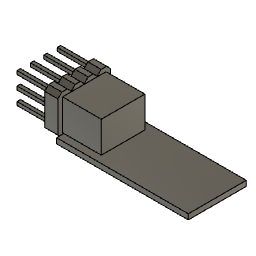
_FS2A Receiver.9ec7e849-6926-4f4f-884d-18c81e3adff5 (Autodesk Fusion 360 design; units mm, degrees)
Autodesk Fusion 360 part; units mm, degrees
sketch "Sketch1" plane through (0, 0, 0) normal (0, 0, 1) x (1, 0, 0)
  line L0 (-12.5, 5.5) -> (12.5, 5.5)
  line L1 (12.5, 5.5) -> (12.5, -5.5)
  line L2 (12.5, -5.5) -> (-12.5, -5.5)
  line L3 (-12.5, -5.5) -> (-12.5, 5.5)
  line L4 (-12.5, 5.5) -> (12.5, -5.5) construction
  line L5 (12.5, 5.5) -> (-12.5, -5.5) construction
  line L6 (-12.5, 5.5) -> (-21.5, 5.5) construction
  line L7 (-21.5, 5.5) -> (-21.5, -5.5) construction
  line L8 (-21.5, -5.5) -> (-12.5, -5.5) construction
  dimension "d1" = 11
  dimension "d2" = 25
  dimension "d5" = 34
  constraint horizontal L0
  constraint vertical L1
  constraint horizontal L2
  constraint vertical L3
  constraint coincident origin L5
  constraint coincident origin L4
  constraint perpendicular L3 L6
  constraint perpendicular L2 L7
  constraint perpendicular L3 L8
  measures "d1" distance of L0.start L2.end
  measures "d2" distance of L0.start L0.end
  measures "d5" distance of L1 L7
extrude "Extrude1" add sketch "Sketch1" along normal blind 1 makes body 1
sketch "Sketch2" plane through (0, 0, 0) normal (0, 1, 0) x (1, 0, 0)
  line L0 (-15.25, -7.75) -> (-12.75, -7.75)
  line L1 (-12.75, -7.75) -> (-12.75, -0.31)
  line L2 (-12.75, -0.31) -> (-15.25, -0.31)
  line L3 (-15.25, -0.31) -> (-15.25, -7.75)
  point P0 (12.5, 0)
  dimension "d6" = 2.5
  dimension "d7" = 7.44
  dimension "d8" = 7.75
  dimension "d9" = 27.75
  constraint horizontal L0
  constraint perpendicular L0 L1
  constraint perpendicular L1 L2
  constraint perpendicular L0 L3
  constraint coincident L0.start L3.end
  measures "d6" distance of L0.start L0.end
  measures "d7" distance of L2.end L0.start
  measures "d8" distance of origin L0
  measures "d9" distance of L3 P0
extrude "Extrude2" add sketch "Sketch2" along normal mid plane 10 separate body makes body 2
sketch "Sketch3" plane through (-15.25, 0, 0) normal (-1, 0, 0) x (0, -1, 0)
  line L0 (5, 7.75) -> (-5, 7.75)
  line L1 (-5, 7.75) -> (-5, 0.31)
  line L2 (-5, 0.31) -> (5, 0.31)
  line L3 (5, 0.31) -> (5, 7.75)
  line L4 (-4.15, 6.9) -> (-3.5, 6.9)
  line L5 (-3.5, 6.9) -> (-3.5, 6.25)
  line L6 (-3.5, 6.25) -> (-4.15, 6.25)
  line L7 (-4.15, 6.25) -> (-4.15, 6.9)
  line L8 (-1.61, 6.9) -> (-0.96, 6.9)
  line L9 (-0.96, 6.9) -> (-0.96, 6.25)
  line L10 (-0.96, 6.25) -> (-1.61, 6.25)
  line L11 (-1.61, 6.25) -> (-1.61, 6.9)
  line L12 (0.93, 6.9) -> (1.58, 6.9)
  line L13 (1.58, 6.9) -> (1.58, 6.25)
  line L14 (1.58, 6.25) -> (0.93, 6.25)
  line L15 (0.93, 6.25) -> (0.93, 6.9)
  line L16 (3.47, 6.9) -> (4.12, 6.9)
  line L17 (4.12, 6.9) -> (4.12, 6.25)
  line L18 (4.12, 6.25) -> (3.47, 6.25)
  line L19 (3.47, 6.25) -> (3.47, 6.9)
  line L20 (-4.15, 4.36) -> (-3.5, 4.36)
  line L21 (-3.5, 4.36) -> (-3.5, 3.71)
  line L22 (-3.5, 3.71) -> (-4.15, 3.71)
  line L23 (-4.15, 3.71) -> (-4.15, 4.36)
  line L24 (-1.61, 4.36) -> (-0.96, 4.36)
  line L25 (-0.96, 4.36) -> (-0.96, 3.71)
  line L26 (-0.96, 3.71) -> (-1.61, 3.71)
  line L27 (-1.61, 3.71) -> (-1.61, 4.36)
  line L28 (0.93, 4.36) -> (1.58, 4.36)
  line L29 (1.58, 4.36) -> (1.58, 3.71)
  line L30 (1.58, 3.71) -> (0.93, 3.71)
  line L31 (0.93, 3.71) -> (0.93, 4.36)
  line L32 (3.47, 4.36) -> (4.12, 4.36)
  line L33 (4.12, 4.36) -> (4.12, 3.71)
  line L34 (4.12, 3.71) -> (3.47, 3.71)
  line L35 (3.47, 3.71) -> (3.47, 4.36)
  line L36 (-4.15, 1.82) -> (-3.5, 1.82)
  line L37 (-3.5, 1.82) -> (-3.5, 1.17)
  line L38 (-3.5, 1.17) -> (-4.15, 1.17)
  line L39 (-4.15, 1.17) -> (-4.15, 1.82)
  line L40 (-1.61, 1.82) -> (-0.96, 1.82)
  line L41 (-0.96, 1.82) -> (-0.96, 1.17)
  line L42 (-0.96, 1.17) -> (-1.61, 1.17)
  line L43 (-1.61, 1.17) -> (-1.61, 1.82)
  line L44 (0.93, 1.82) -> (1.58, 1.82)
  line L45 (1.58, 1.82) -> (1.58, 1.17)
  line L46 (1.58, 1.17) -> (0.93, 1.17)
  line L47 (0.93, 1.17) -> (0.93, 1.82)
  line L48 (3.47, 1.82) -> (4.12, 1.82)
  line L49 (4.12, 1.82) -> (4.12, 1.17)
  line L50 (4.12, 1.17) -> (3.47, 1.17)
  line L51 (3.47, 1.17) -> (3.47, 1.82)
  line L52 (-5, 7) -> (-4.25, 7.75)
  line L53 (-3.21, 7.75) -> (-2.46, 7)
  line L54 (-2.46, 7) -> (-1.71, 7.75)
  line L55 (-0.75, 7.75) -> (0, 7)
  line L56 (0, 7) -> (0.7523, 7.7523)
  line L57 (1.71, 7.75) -> (2.46, 7)
  line L58 (2.46, 7) -> (3.21, 7.75)
  line L59 (4.25, 7.75) -> (5, 7)
  line L60 (-5, 7) -> (5, 7) construction
  line L61 (-5, 7) -> (-5, 8.8118)
  line L62 (-5, 8.8118) -> (5, 8.8118)
  line L63 (5, 8.8118) -> (5, 7)
  line L64 (-4.25, 7.75) -> (-3.21, 7.75)
  line L65 (-1.71, 7.75) -> (-0.75, 7.75)
  line L66 (0.7523, 7.7523) -> (1.71, 7.75)
  line L67 (3.21, 7.75) -> (4.25, 7.75)
  line L68 (-5, 1.06) -> (5, 1.06) construction
  line L69 (-5, 1.06) -> (-5, -0.1236)
  line L70 (-5, -0.1236) -> (5, -0.1236)
  line L71 (5, -0.1236) -> (5, 1.06)
  line L72 (5, 1.06) -> (4.25, 0.31)
  line L73 (4.25, 0.31) -> (3.21, 0.31)
  line L74 (3.21, 0.31) -> (2.46, 1.06)
  line L75 (2.46, 1.06) -> (1.71, 0.31)
  line L76 (1.71, 0.31) -> (0.75, 0.31)
  line L77 (0.75, 0.31) -> (0, 1.06)
  line L78 (0, 1.06) -> (-0.75, 0.31)
  line L79 (-0.75, 0.31) -> (-1.71, 0.31)
  line L80 (-1.71, 0.31) -> (-2.46, 1.06)
  line L81 (-2.46, 1.06) -> (-3.21, 0.31)
  line L82 (-3.21, 0.31) -> (-4.25, 0.31)
  line L83 (-4.25, 0.31) -> (-5, 1.06)
  line L84 (-4.15, 6.9) -> (4.12, 6.9)
  line L85 (4.12, 6.9) -> (4.12, 1)
  line L86 (4.12, 1) -> (-4.15, 1)
  line L87 (-4.15, 1) -> (-4.15, 6.9)
  line L88 (-5.5, 1) -> (5.5, 1)
  dimension "d12" = 0.65
  dimension "d13" = 0.65
  dimension "d16" = 2.54
  dimension "d17" = -2.54
  dimension "d18" = 0.85
  dimension "d19" = 0.85
  dimension "d20" = 0.75
  dimension "d21" = 90
  dimension "d22" = 45
  dimension "d23" = 90
  dimension "d24" = 90
  dimension "d25" = 45
  dimension "d26" = 2.54
  dimension "d27" = 2.54
  dimension "d28" = 0.75
  constraint horizontal L4
  constraint vertical L5
  constraint horizontal L6
  constraint vertical L7
  constraint coincident L1 L52.start
  constraint coincident L0 L52.end
  constraint coincident L0 L53.start
  constraint coincident L0 L54.end
  constraint coincident L0 L55.start
  constraint coincident L0 L57.start
  constraint coincident L0 L58.end
  constraint coincident L0 L59.start
  constraint coincident L3 L59.end
  constraint horizontal L60
  constraint perpendicular L60 L61
  constraint perpendicular L3 L62
  constraint perpendicular L60 L63
  constraint coincident L53.end L60
  constraint coincident L55.end L60
  constraint coincident L57.end L60
  constraint vertical origin L55.end
  constraint parallel L52 L54
  constraint parallel L54 L56
  constraint parallel L56 L58
  constraint coincident L1 L68.start
  constraint coincident L3 L68.end
  constraint perpendicular L3 L68
  constraint perpendicular L68 L69
  constraint perpendicular L3 L70
  constraint perpendicular L68 L71
  constraint coincident L2 L72.end
  constraint coincident L2 L73.end
  constraint parallel L2 L73
  constraint coincident L68 L74.end
  constraint coincident L2 L75.end
  constraint parallel L72 L75
  constraint coincident L2 L76.end
  constraint parallel L2 L76
  constraint midpoint L68 L77.end
  constraint coincident L2 L78.end
  constraint perpendicular L77 L78
  constraint coincident L2 L79.end
  constraint parallel L2 L79
  constraint coincident L68 L80.end
  constraint coincident L2 L81.end
  constraint perpendicular L80 L81
  constraint coincident L2 L82.end
  constraint parallel L2 L82
  constraint vertical L53.end L80.end
  constraint vertical L57.end L74.end
  constraint parallel L59 L83
  constraint parallel L80 L83
  constraint parallel L77 L80
  constraint parallel L74 L77
  constraint parallel L52 L72
  constraint horizontal L84
  constraint vertical L85
  constraint horizontal L86
  constraint vertical L87
  constraint coincident L86.end L88
  measures "d12" distance of L4.start L4.end
  measures "d13" distance of L4.start L6.end
  measures "d18" distance of L0 L4
  measures "d19" distance of L1 L7
  measures "d20" distance of L0 L60
  measures "d21" angle of L55 L56
  measures "d22" angle of L52 L61
  measures "d23" angle of L53 L54
  measures "d24" angle of L57 L58
  measures "d25" angle of L59 L63
  measures "d26" distance of L52.start L53.end
  measures "d27" distance of L57.end L59.end
  measures "d28" distance of L2 L68
extrude "Extrude3" cut sketch "Sketch3" against normal blind 3 contours L0 L3 L59 L63 | L0 L56 L61 L62 L63 L64 L65 L66 L67 | L0 L57 L58 | L3 L71 L72 L88 | L2 L3 L71 L72 L88 | L0 L1 L52 L61 | L0 L55 L56 | L2 L69 L70 L71 L73 L76 L79 L82 | L2 L74 L75 L86 L88 | L74 L75 L86 L88 | L0 L53 L54 | L1 L69 L83 L88 | L1 L2 L69 L83 L88 | L2 L77 L78 L86 L88 | L77 L78 L86 L88 | L2 L80 L81 L86 L88 | L80 L81 L86 L88 bodies 2
extrude "Extrude4" add sketch "Sketch3" along normal blind 6.14 contours L48 L49 L50 L51 L85 | L32 L33 L34 L35 L85 | L36 L37 L38 L39 L87 | L16 L17 L18 L19 L84 L85 | L20 L21 L22 L23 L87 | L12 L13 L14 L15 L84 | L4 L5 L6 L7 L84 L87 | L8 L9 L10 L11 L84 | L24 L25 L26 L27 | L28 L29 L30 L31 | L40 L41 L42 L43 | L44 L45 L46 L47 bodies 2
extrude "Extrude5" add sketch "Sketch3" against normal blind 7.36 from surface at -2.5 contours L5 L6 L9 L10 L11 L13 L14 L15 L18 L19 L20 L21 L22 L32 L34 L35 L36 L37 L38 L48 L50 L51 L74 L75 L77 L78 L80 L81 L84 L85 L86 L87 L88 | L48 L49 L50 L51 L85 | L74 L75 L86 L88 | L32 L33 L34 L35 L85 | L77 L78 L86 L88 | L80 L81 L86 L88 | L36 L37 L38 L39 L87 | L16 L17 L18 L19 L84 L85 | L20 L21 L22 L23 L87 | L12 L13 L14 L15 L84 | L4 L5 L6 L7 L84 L87 | L8 L9 L10 L11 L84 | L24 L25 L26 L27 | L28 L29 L30 L31 | L40 L41 L42 L43 | L44 L45 L46 L47 bodies 1 2
equation "d28 = d20"
